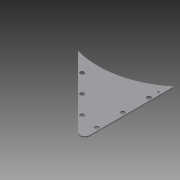
# Autodesk Inventor part: SolarPanel_A
Saved by Autodesk Inventor 2014 SP1 (Build 180222100, 222)
## iProperties
Created: 2015-03-29
Part Number: SolarPanel_A
Material: Generic
Document SubType Name: Modeling
Designer: Erin
Density: 1 g/cm^3
Appearance: Default
Author: Erin
Autodesk Inventor part; units mm, degrees
ref_plane "YZ Plane" through (0, 0, 0) normal (1, 0, 0) x (0, 1, 0)
ref_plane "XZ Plane" through (0, 0, 0) normal (0, 1, 0) x (-1, 0, 0)
ref_plane "XY Plane" through (0, 0, 0) normal (0, 0, 1) x (1, 0, 0)
sketch "Sketch1" plane through (0, 0, 0) normal (0, 0, 1) x (1, 0, 0)
  line L0 (5.692, 95.6468) -> (5.692, 8.2889)
  line L1 (14.2275, 4.7534) -> (87.4433, 77.9691)
  arc A0 (5.692, 95.6468) -> (87.4433, 77.9691) centre (63.3991, 164.6459) ccw
  line L2 (59.8725, 27.771) -> (44.3162, 43.3273) construction
  circle A1 centre (46.4375, 41.206) radius 2.25
  circle A2 centre (27.3392, 22.1077) radius 2.25
  circle A3 centre (65.523, 60.2915) radius 2.25
  circle A4 centre (8.692, 18.6468) radius 2.25
  circle A5 centre (8.692, 45.6468) radius 2.25
  circle A6 centre (8.692, 72.6468) radius 2.25
  arc A7 (5.692, 8.2889) -> (14.2275, 4.7534) centre (10.692, 8.2889) ccw
  line L3 (0, -29.262) -> (0, 157.4073) construction
  line L4 (8.692, 99.7724) -> (8.692, -5.6931) construction
  line L5 (0.8124, -4.4191) -> (92.0626, 86.8311) construction
  circle A8 centre (8.692, 82.6468) radius 1
  point P0 (0, 0)
  dimension "d0" = 4.5
  dimension "d1" = 4.5
  dimension "d2" = 4.5
  dimension "d3" = 5
  dimension "d4" = 3
  dimension "d5" = 3
  dimension "d8" = 2
  dimension "d9" = 10
  constraints: 12 end point, 9 centre point, 7 point on line, 4 point on circle, 2 parallel, 2 tangent, 2 vertical, 1 midpoint, 1 perpendicular, 2 other
  measures "d0" diameter of A1
  measures "d1" diameter of A2
  measures "d2" diameter of A3
  measures "d3" radius of A7
  measures "d4" distance between parallel lines of L0 L4
  measures "d5" distance between parallel lines of L5 L1
  measures "d8" diameter of A8
  measures "d9" distance of A8.centre A6.centre
extrude "Extrusion1" add sketch "Sketch1" along normal blind 1
mirror "Mirror1" about plane through (0, 0, 0) normal (1, 0, 0) remove original yes
body "Solid1"
